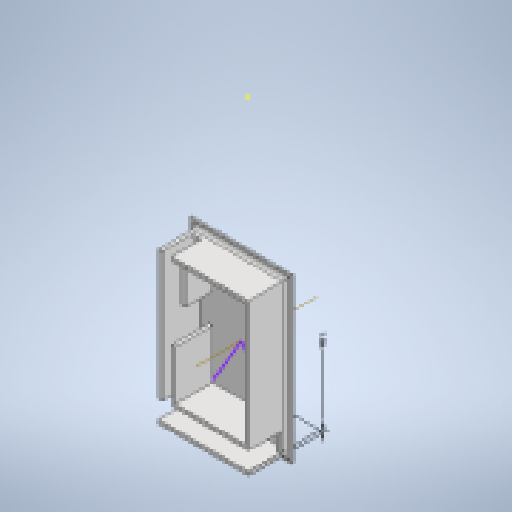
# Autodesk Inventor part: Base4Baterias
Saved by Autodesk Inventor 2024 (Build 280153000, 153)
## iProperties
Created: 2024-07-14
Part Number: Base4Baterias
Material: Genérico
Document SubType Name: Modeling
Designer: sergi
Density: 1 g/cm^3
Appearance: Valor por defecto
Author: sergi
Autodesk Inventor part; units mm, degrees
ref_plane "YZ Plane" through (0, 0, 0) normal (1, 0, 0) x (0, 1, 0)
ref_plane "XZ Plane" through (0, 0, 0) normal (0, 1, 0) x (-1, 0, 0)
ref_plane "Plano de trabajo1" through (0, 0, 0) normal (0, 0, 1) x (1, 0, 0)
sketch "Boceto1" plane through (0, 0, 0) normal (0, 0, 1) x (1, 0, 0)
  line L0 (0.4509, -110.4895) -> (0.451, -110.4898) projected
  line L1 (0.4512, -110.4895) -> (0.4509, -110.4895) projected
  line L2 (-0.0742, -109.5793) -> (0.4512, -110.4895) projected
  line L3 (-0.5999, -110.4893) -> (0.1885, -110.0344)
  line L4 (0.4512, -110.4895) -> (-0.3337, -110.0363)
  line L5 (0.4512, -110.4895) -> (-0.5999, -110.4895)
  line L6 (-0.5999, -110.4895) -> (-0.0743, -109.5792)
  line L7 (-0.0743, -109.5792) -> (0.4512, -110.4895)
  line L8 (-95.0743, -55.3377) -> (94.9257, -55.3377)
  line L9 (94.9257, -55.3377) -> (-0.0743, -219.8826)
  line L10 (-0.0743, -219.8826) -> (-95.0743, -55.3377)
  point P0 (0, 0)
  point P1 (-0.0743, -110.186)
  point P2 (-0.0743, -110.186)
  point P3 (0.1885, -110.0344)
  dimension "d0" = 190
  constraints: 16 end point, 3 point on line, 1 coincident, 1 horizontal, 1 midpoint, 14 other
  measures "d0" distance of L8.start L8.end
extrude "Extrusión1" add sketch "Boceto1" along normal blind 1.5 contours L2 L3 L6 | L2 L4 L3 | L3 L4 L5 | L8 L9 L10
fillet "Empalme1" radius 30 3 edges at (-95.0743, -55.3377, 0.75) (94.9257, -55.3377, 0.75) (-0.0743, -219.8826, 0.75)
sketch "Boceto2" plane through (0, 0, 1.5) normal (0, 0, 1) x (1, 0, 0)
  line L0 (25.9064, -174.8826) -> (68.9449, -100.3377) projected
  line L1 (42.9642, -55.3377) -> (-43.1128, -55.3377) projected
  line L2 (-69.0936, -100.3377) -> (-26.0551, -174.8826) projected
  line L3 (0.4512, -110.4895) -> (0.1885, -110.0344) projected
  line L4 (0.1885, -110.0344) -> (0.1885, -110.0344) projected
  line L5 (0.1885, -110.0344) -> (0.4512, -110.4895) projected
  line L6 (-0.0743, -219.8826) -> (94.9257, -55.3377) projected
  line L7 (-0.0743, -219.8826) -> (-0.0743, -55.3377)
  line L8 (-18.8243, -77.186) -> (18.6757, -77.186)
  line L9 (18.6757, -77.186) -> (18.6757, -143.186)
  line L10 (18.6757, -143.186) -> (-18.8243, -143.186)
  line L11 (-18.8243, -143.186) -> (-18.8243, -77.186)
  line L12 (-18.8243, -77.186) -> (18.6757, -143.186) construction
  line L13 (18.6757, -77.186) -> (-18.8243, -143.186) construction
  line L14 (-20.8243, -75.186) -> (20.6757, -75.186)
  line L15 (20.6757, -75.186) -> (20.6757, -145.186)
  line L16 (20.6757, -145.186) -> (-20.8243, -145.186)
  line L17 (-20.8243, -145.186) -> (-20.8243, -75.186)
  line L18 (94.9257, -55.3377) -> (57.0834, -77.186)
  arc A0 (-26.0551, -174.8826) -> (25.9064, -174.8826) centre (-0.0743, -159.8826) ccw projected
  arc A1 (68.9449, -100.3377) -> (42.9642, -55.3377) centre (42.9642, -85.3377) ccw projected
  arc A2 (-43.1128, -55.3377) -> (-69.0936, -100.3377) centre (-43.1128, -85.3377) ccw projected
  point P0 (0, 0)
  dimension "d4" = 37.5
  dimension "d5" = 66
  dimension "d6" = 2
  constraints: 24 end point, 4 parallel, 2 perpendicular, 1 horizontal, 1 midpoint, 1 point on line, 3 other
  measures "d4" distance of L9.end L10.end
  measures "d5" distance of L8.end L9.end
  measures "d6" distance between parallel lines of L11 L17
extrude "Extrusión2" add sketch "Boceto2" along normal blind 20.25 contours L16 L17 L14 L7 L8 L11 L10 | L7 L10 L9 L8 L14 L15 L16
sketch "Boceto3" plane through (-20.8243, -145.186, 21.75) normal (-1, 0, 0) x (0, 0, 1)
  line L0 (-20.25, 0) -> (0, 0) projected
  line L1 (0, 70) -> (0, 0) projected
  line L2 (-20.25, 70) -> (0, 70) projected
  line L3 (0, 70) -> (-18.05, 70)
  line L4 (-18.05, 70) -> (-18.05, 44.7)
  line L5 (-18.05, 44.7) -> (0, 44.7)
  line L6 (0, 44.7) -> (0, 70)
  line L7 (-20.25, 0) -> (-20.25, 70) projected
  line L8 (0, 0) -> (-17, 0)
  line L9 (-17, 0) -> (-17, 28.6)
  line L10 (-17, 28.6) -> (0, 28.6)
  line L11 (0, 28.6) -> (0, 0)
  line L12 (-18.05, 44.7) -> (-20.25, 44.7)
  line L13 (-17, 28.6) -> (-20.25, 28.6)
  point P0 (-21.75, 145.186)
  point P1 (0, 28.6)
  point P2 (0, 44.7)
  dimension "d10" = 18.05
  dimension "d11" = 25.3
  dimension "d12" = 17
  dimension "d13" = 28.6
  constraints: 20 end point, 4 parallel, 4 perpendicular, 2 horizontal, 2 point on line
  measures "d10" distance of L5.end L4.end
  measures "d11" distance of L3.end L4.end
  measures "d12" distance of L9.end L10.end
  measures "d13" distance of L8.end L9.end
sketch "Boceto4" plane through (0, 0, 1.5) normal (0, 0, 1) x (1, 0, 0)
  line L0 (20.6757, -145.186) -> (20.6757, -75.186) projected
  line L1 (20.6757, -75.186) -> (-20.8243, -75.186) projected
  line L2 (-20.8243, -75.186) -> (-20.8243, -145.186) projected
  line L3 (-20.8243, -145.186) -> (20.6757, -145.186) projected
  line L4 (18.6757, -143.186) -> (-18.8243, -143.186) projected
  line L5 (-18.8243, -143.186) -> (-18.8243, -77.186) projected
  line L6 (-18.8243, -77.186) -> (18.6757, -77.186) projected
  line L7 (18.6757, -77.186) -> (18.6757, -143.186) projected
  line L8 (-25.8243, -75.186) -> (-25.8243, -145.186)
  line L9 (-25.8243, -75.186) -> (-27.8243, -75.186)
  line L10 (-27.8243, -75.186) -> (-27.8243, -156.986)
  line L11 (-27.8243, -145.186) -> (-25.8243, -145.186)
  line L12 (-20.8243, -154.986) -> (-20.8243, -156.986)
  line L13 (-20.8243, -156.986) -> (20.6757, -156.986)
  line L14 (20.6757, -156.986) -> (20.6757, -154.986)
  line L15 (20.6757, -154.986) -> (-20.8243, -154.986)
  line L16 (-20.8243, -156.986) -> (-27.8243, -156.986)
  line L17 (-25.8243, -145.186) -> (-25.8243, -154.986)
  line L18 (-25.8243, -154.986) -> (-20.8243, -154.986)
  line L19 (20.6757, -145.186) -> (20.6757, -154.986)
  line L20 (20.6757, -145.186) -> (18.6757, -145.186)
  line L21 (18.6757, -145.186) -> (18.6757, -154.986)
  line L22 (-20.8243, -75.186) -> (-25.8243, -75.186)
  line L23 (-20.8243, -75.186) -> (-20.8243, -77.186)
  line L24 (-20.8243, -77.186) -> (-25.8243, -77.186)
  point P0 (0, 0)
  dimension "d19" = 2
  dimension "d22" = 2
  dimension "d23" = 2
  constraints: 34 end point, 7 point on line, 6 perpendicular, 3 horizontal, 2 vertical, 1 parallel
  measures "d19" distance of L13.end L14.end
  measures "d22" distance of L0.start L20.end
  measures "d23" distance of L1.end L23.end
extrude "Extrusión3" add sketch "Boceto4" along normal blind 20.25 contours L19 L15 L21 L3 | L14 L13 L12 L15 | L2 L24 L8 L22 | L8 L11 L10 L9 | L12 L16 L10 L11 L17 L18
extrude "Extrusión4" cut sketch "Boceto3" against normal up to surface (2 mm away) contours L7 L12 L5 L1 L10 L13
sketch "Boceto5" plane through (-20.8243, -77.186, 1.5) normal (-1, 0, 0) x (0, 0, 1)
  line L0 (0, 0) -> (15, 0)
  line L1 (15, 0) -> (15, -23.3)
  line L2 (15, -23.3) -> (0, -23.3)
  line L3 (0, -23.3) -> (0, 0)
  line L4 (0, -23.3) -> (20.25, -23.3) projected
  line L5 (20.25, 0) -> (20.25, -23.3) projected
  line L6 (20.25, 0) -> (0, 0) projected
  line L7 (0, -23.3) -> (0, 0) projected
  point P0 (-1.5, 77.186)
  point P1 (15, -23.3)
  dimension "d26" = 15
  dimension "d27" = 23.3
  constraints: 8 end point, 2 parallel, 1 horizontal, 1 perpendicular
  measures "d26" distance of L1.end L2.end
  measures "d27" distance of L0.end L1.end
extrude "Extrusión5" cut sketch "Boceto5" against normal up to surface (2 mm away) contours L6 L5 L4 L1
sketch "Boceto6" plane through (-25.8243, -154.986, 1.5) normal (1, 0, 0) x (0, 0, -1)
  line L0 (0, 9.8) -> (-20.25, 9.8) projected
  line L1 (0, 77.8) -> (0, 0) projected
  line L2 (0, 77.8) -> (-20.25, 77.8) projected
  line L3 (-20.25, 0) -> (-20.25, 77.8) projected
  line L4 (0, 0) -> (-20.25, 0) projected
  line L5 (0, 0) -> (-11.6, 0)
  line L6 (-11.6, 0) -> (-11.6, 9.8)
  line L7 (-11.6, 9.8) -> (0, 9.8)
  line L8 (0, 9.8) -> (0, 0)
  point P0 (1.5, 154.986)
  dimension "d30" = 11.6
  constraints: 8 end point, 2 parallel, 1 horizontal, 1 perpendicular, 1 point on line
  measures "d30" distance of L6.end L7.end
extrude "Extrusión6" cut sketch "Boceto6" against normal up to surface (2 mm away) contours L1 L4 L6 L0 | L6 L4 L3 L0
sketch "Boceto7" plane through (-18.8243, -77.186, 1.5) normal (0, -1, 0) x (1, 0, 0)
  line L0 (-2, 0) -> (-7, 0) projected
  line L1 (-2, 15) -> (-2, 0) projected
  line L2 (-2, 15) -> (0, 15) projected
  line L3 (0, 0) -> (0, 15) projected
  line L4 (37.5, 0) -> (0, 0) projected
  line L5 (37.5, 0) -> (37.5, 20.25) projected
  line L6 (-7, 20.25) -> (37.5, 20.25) projected
  line L7 (-7, 0) -> (-7, 20.25) projected
  line L8 (-2, 15) -> (-2, 20.25)
  line L9 (-7, 0) -> (-2, 0)
  line L10 (-2, 0) -> (-2, 4)
  line L11 (-2, 4) -> (-7, 4)
  line L12 (-7, 4) -> (-7, 0)
  point P0 (18.8243, -1.5)
  point P1 (-7, 4)
  dimension "d35" = 4
  constraints: 10 end point, 2 parallel, 2 point on line, 1 horizontal, 1 perpendicular, 1 vertical
  measures "d35" distance of L10.end L9.end
extrude "Extrusión7" cut sketch "Boceto7" against normal up to surface (2 mm away) contours L11 L7 L6 L8 L1
ref_plane "Plano de trabajo2" through (0, 0, 1.5) normal (0, 0, 1) x (1, 0, 0)
split "Dividir1" plane through (0, 0, 1.5) removes the side toward (0, 0, -1)
sketch "Boceto8" plane through (20.6757, -156.986, 1.5) normal (0, 0, -1) x (-1, 0, 0)
  line L0 (48.5, 0) -> (0, 0) projected
  line L1 (24.2796, 40.9499) -> (48.5, 0)
  line L2 (48.5, 81.8) -> (48.5, 11.8) projected
  line L3 (0, 0) -> (0, 81.8) projected
  line L4 (24.2796, 40.9499) -> (0, 0)
  point P0 (20.6757, 156.986)
  constraints: 4 end point
ref_plane "Plano de trabajo3" through (-3.5743, -110.9343, 1.5) normal (0, 0, 1) x (1, 0, 0)
sketch "Boceto9" plane through (20.6757, -156.986, 21.75) normal (1, 0, 0) x (0, 0, -1)
  line L0 (20.25, 81.8) -> (20.25, 0) projected
  line L1 (20.25, 81.8) -> (0, 81.8) projected
  line L2 (0, 0) -> (0, 81.8) projected
  line L3 (20.25, 0) -> (0, 0) projected
  line L4 (20.25, 2) -> (20.25, 11.8) projected
  line L5 (20.25, 2) -> (0, 2) projected
  line L6 (0, 11.8) -> (0, 2) projected
  line L7 (20.25, 11.8) -> (0, 11.8) projected
  line L8 (0, 2) -> (20.25, 11.8)
  line L9 (17.125, 2.15) -> (3.125, 2.15)
  line L10 (3.125, 2.15) -> (3.125, 11.65)
  line L11 (3.125, 11.65) -> (17.125, 11.65)
  line L12 (17.125, 11.65) -> (17.125, 2.15)
  line L13 (17.125, 2.15) -> (3.125, 11.65) construction
  line L14 (3.125, 2.15) -> (17.125, 11.65) construction
  line L15 (3.125, 2) -> (17.125, 2)
  line L16 (17.125, 2) -> (17.125, 11.8)
  line L17 (17.125, 11.8) -> (3.125, 11.8)
  line L18 (3.125, 11.8) -> (3.125, 2)
  point P0 (21.75, 156.986)
  point P1 (12.7514, 35.7395)
  point P2 (10.125, 6.9)
  point P3 (3.125, 11.65)
  point P4 (3.125, 2.15)
  point P5 (3.125, 11.65)
  point P6 (3.125, 2.15)
  point P7 (17.125, 2.15)
  point P8 (17.125, 10.2877)
  point P9 (17.125, 11.65)
  dimension "d43" = 14
  dimension "d44" = 9.5
  constraints: 22 end point, 4 parallel, 3 midpoint, 2 horizontal, 2 perpendicular, 2 point on line, 1 other
  measures "d43" distance of L10.end L11.end
  measures "d44" distance of L9.end L10.end
extrude "Extrusión8" cut sketch "Boceto9" against normal up to surface (2 mm away) contours L16 L11 L18 L7 | L12 L9 L10 L8 | L8 L10 L11 L12 | L7 L18 L10 L8 L2 | L5 L18 L9 L16 | L10 L18 L5 L8
sketch "Boceto10" plane through (20.6757, -156.986, 1.5) normal (0, 0, -1) x (-1, 0, 0)
  line L0 (49, 82) -> (0, 82)
  line L1 (0, 82) -> (0, 0)
  line L2 (0, 0) -> (49, 0)
  line L3 (49, 0) -> (49, 82)
  line L4 (52, 85) -> (-3, 85)
  line L5 (-3, 85) -> (-3, -3)
  line L6 (-3, -3) -> (52, -3)
  line L7 (52, -3) -> (52, 85)
  point P0 (20.6757, 156.986)
  dimension "d47" = 3
  constraints: 16 end point, 4 parallel, 2 perpendicular, 1 horizontal, 3 other
  measures "d47" distance between parallel lines of L3 L7
extrude "Extrusión9" add sketch "Boceto10" along normal blind 1 contours L3 L2 L1 L0 | L7 L6 L5 L4
fillet "Empalme3" radius 2 5 edges at (-27.8243, -110.186, 1.5) (-27.8243, -155.986, 1.5) (-3.5743, -156.986, 1.5) (20.6757, -116.086, 1.5) (-3.5743, -75.186, 1.5)
